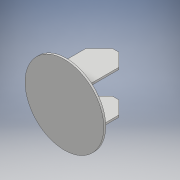
# Autodesk Inventor part: Bras principal
Saved by Autodesk Inventor 2018 (Build 220112000, 112)
## iProperties
Created: 2018-03-19
Part Number: Bras principal
Material: Générique
Document SubType Name: Modeling
Designer: Youri
Density: 1 g/cm^3
Appearance: Par défaut
Author: Youri
Autodesk Inventor part; units mm, degrees
ref_plane "YZ Plane" through (0, 0, 0) normal (1, 0, 0) x (0, 1, 0)
ref_plane "XZ Plane" through (0, 0, 0) normal (0, 1, 0) x (-1, 0, 0)
ref_plane "XY Plane" through (0, 0, 0) normal (0, 0, 1) x (1, 0, 0)
sketch "Esquisse1" plane through (0, 0, 0) normal (0, 1, 0) x (-1, 0, 0)
  circle A0 centre (0, 0) radius 60
  dimension "d0" = 120
  constraints: 1 centre point, 1 coincident
  measures "d0" diameter of A0
extrude "Extrusion1" add sketch "Esquisse1" along normal blind 3
sketch "Esquisse2" plane through (0, 3, 0) normal (0, 1, 0) x (1, 0, 0)
  line L0 (-25, -33) -> (25, -33)
  line L1 (25, -33) -> (25, -30)
  line L2 (25, -30) -> (-25, -30)
  line L3 (-25, -30) -> (-25, -33)
  line L4 (-25, 33) -> (25, 33)
  line L5 (25, 33) -> (25, 30)
  line L6 (25, 30) -> (-25, 30)
  line L7 (-25, 30) -> (-25, 33)
  point P0 (0, 0)
  dimension "d3" = 50
  dimension "d4" = 50
  dimension "d5" = 30
  dimension "d7" = 30
  dimension "d8" = 3
  dimension "d9" = 3
  dimension "d10" = 25
  constraints: 16 end point, 4 parallel, 2 horizontal, 2 perpendicular, 2 point on line
  measures "d3" distance of L1.end L2.end
  measures "d4" distance of L5.end L6.end
  measures "d5" distance from line of point (0, 0) L2
  measures "d7" distance from line of point (0, 0) L6
  measures "d8" distance of L2.end L0.start
  measures "d9" distance of L4.end L5.end
  measures "d10" horizontal distance of point (0, 0) L2.end
extrude "Extrusion2" add sketch "Esquisse2" along normal blind 75
chamfer "Chanfrein1" distance 20 angle 45 4 edges at (25, 78, 31.5) (25, 78, -31.5) (-25, 78, -31.5) (-25, 78, 31.5)
